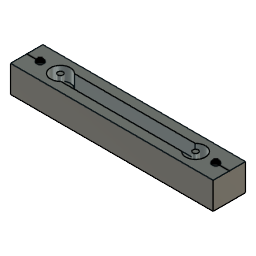
hexbug_5.5cm_mold_final (Autodesk Fusion 360 design; units mm, degrees)
Autodesk Fusion 360 part; units mm, degrees
note: some values were not read from the file. Set by a fixed rule: which sketch regions a step uses.
sketch "Sketch1" plane through (0, 0, 0) normal (0, 0, 1) x (1, 0, 0)
  line L0 (0, 0) -> (-55, 0)
  line L1 (-55, 0) -> (-55, -12)
  line L2 (-55, -12) -> (0, -12)
  line L3 (0, -12) -> (0, 0)
  dimension "d1" = 12
  dimension "d2" = 55
  constraint horizontal L0
  constraint vertical L1
  constraint horizontal L2
  constraint vertical L3
  constraint coincident L0.start L3.end
  measures "d1" distance of L0.start L2.end
  measures "d2" distance of L0.start L0.end
extrude "Extrude1" add sketch "Sketch1" along normal blind 10 makes body 1
sketch "Sketch2" plane through (0, 0, 10) normal (0, 0, 1) x (-1, 0, 0)
  line L0 (0, 12) -> (0, 0)
  line L1 (0, 0) -> (55, 0)
  line L2 (55, 0) -> (55, 12)
  line L3 (55, 12) -> (0, 12)
  line L4 (0, 6) -> (55, 6)
  line L5 (27.5, 12) -> (27.5, 0)
  line L6 (27.5, 6) -> (2.5, 6)
  line L7 (27.5, 6) -> (52.5, 6)
  circle A0 centre (2.5, 6) radius 1
  circle A1 centre (52.5, 6) radius 1
  line L8 (2.5, 6) -> (2.5, 3.5)
  line L9 (52.5, 3.5) -> (2.5, 3.5)
  line L10 (2.5, 8.5) -> (52.5, 8.5)
  circle A2 centre (2.5, 6) radius 3.65
  circle A3 centre (52.5, 6) radius 3.65
  dimension "d5" = 25
  dimension "d6" = 25
  dimension "d7" = 2
  dimension "d9" = 2
  dimension "d19" = 7.3
  dimension "d20" = 7.3
  constraint midpoint L0 L4.start
  constraint midpoint L2 L4.end
  constraint midpoint L3 L5.start
  constraint midpoint L1 L5.end
  constraint midpoint L4 L6.start
  constraint perpendicular L0 L6
  constraint perpendicular L5 L7
  constraint coincident L6.end A0.centre
  constraint coincident L7.end A1.centre
  constraint perpendicular L4 L8
  constraint parallel L9 L10
  constraint concentric A0 A2
  measures "d5" distance of L6.start L6.end
  measures "d6" distance of L6.start L7.end
  measures "d7" diameter of A0
  measures "d9" diameter of A1
  measures "d19" diameter of A2
  measures "d20" diameter of A3
extrude "Extrude10" add 1 faces at (-55, -4, 3.3333) along direction (-1, 0, 0) blind 10 on bodies 1 bodies 1
extrude "Extrude11" add 1 faces at (0, -8, 3.3333) along direction (1, 0, 0) blind 10 on bodies 1 bodies 1
sketch "Sketch3" plane through (0, 0, 10) normal (0, 0, 1) x (-1, 0, 0)
  line L0 (-10, 0) -> (65, 0)
  line L1 (65, 0) -> (65, 12)
  line L2 (65, 12) -> (-10, 12)
  line L3 (-10, 12) -> (-10, 0)
  line L4 (-10, 6) -> (-5, 6)
  circle A0 centre (-5, 6) radius 1.25
  line L5 (65, 6) -> (60, 6)
  circle A1 centre (60, 6) radius 1.25
  dimension "d33" = 5
  dimension "d34" = 2.5
  dimension "d35" = 5
  dimension "d36" = 2.5
  constraint midpoint L3 L4.start
  constraint perpendicular L3 L4
  constraint coincident L4.end A0.centre
  constraint midpoint L1 L5.start
  constraint perpendicular L1 L5
  constraint coincident L5.end A1.centre
  measures "d33" distance of L4.start L4.end
  measures "d34" diameter of A0
  measures "d35" distance of L5.start L5.end
  measures "d36" diameter of A1
extrude "Extrude12" add sketch "Sketch3" along normal blind 10 contours L0 L1 L2 L3 | A0 | A1 bodies 1
sketch "Sketch4" plane through (0, -12, 0) normal (0, -1, 0) x (1, 0, 0)
  line L0 (-65, 0) -> (10, 0)
  line L1 (10, 0) -> (10, 20)
  line L2 (10, 20) -> (-65, 20)
  line L3 (-65, 20) -> (-65, 0)
  line L4 (10, 10) -> (-65, 10)
  constraint midpoint L1 L4.start
  constraint midpoint L3 L4.end
split "Split1" by curves path "Sketch4" along L4 bodies 1 makes body 2 at (-15, -8, 20)
extrude "Extrude13" add sketch "Sketch3" along normal blind 2.5 contours A0 | A1 bodies 1
extrude "Extrude14" cut sketch "Sketch2" against normal blind 5 contours L0 L4 L6 A0 A2 | L0 A2 | L0 L4 A0 L8 L9 A2 | L4 L5 L6 L10 A2 | L4 L5 L7 L10 A3 | L4 L6 A0 L8 L9 A2 | L4 L5 L6 L9 A2 | L2 A3 | L2 L4 L7 A1 A3 | L4 L5 L7 L9 A3 | L2 L4 L7 A1 A3 bodies 1
extrude "Extrude16" cut 2 faces at (-60.1522, -5.6121, 12.5) (5.6109, -6.2456, 12.5) along direction (0, 0, -1) blind 2.5 on bodies 1 bodies 1
extrude "Extrude15" [rolled back] along distance 2.5 taper angle 0
hole "Hole1" [rolled back] hole depth 10 hole diameter 9 tip angle 180 csdiameter 18 csangle 90
extrude "Extrude2" [rolled back] along distance 5 taper angle 0
extrude "Extrude3" [rolled back] along distance 5 taper angle 0
extrude "Extrude4" [rolled back] along distance -2 taper angle 0
extrude "Extrude5" [rolled back] along distance -3 taper angle 0
extrude "Extrude6" [rolled back] along distance 5 taper angle 0
extrude "Extrude7" [rolled back] along distance -5 taper angle 0
extrude "Extrude8" [rolled back] along distance -5 taper angle 0
extrude "Extrude9" [rolled back] along distance -2 taper angle 0
hidden bodies 2
